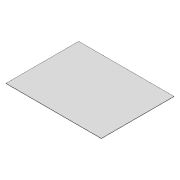
# Autodesk Inventor part: FirewallDiagonal
Saved by Autodesk Inventor 2021 (Build 250183000, 183)
## iProperties
Created: 2020-10-17
Part Number: FirewallDiagonal
Material: Generic
Document SubType Name: Modeling
Designer: PhotonUser
Density: 1 g/cm^3
Appearance: Default
Author: PhotonUser
Autodesk Inventor part; units mm, degrees
ref_plane "YZ Plane" through (0, 0, 0) normal (1, 0, 0) x (0, 1, 0)
ref_plane "XZ Plane" through (0, 0, 0) normal (0, 1, 0) x (-1, 0, 0)
ref_plane "XY Plane" through (0, 0, 0) normal (0, 0, 1) x (1, 0, 0)
sketch "Sketch1" plane through (0, 0, 0) normal (0, 1, 0) x (-1, 0, 0)
  line L0 (284.8412, -112.3127) -> (-273.9588, -112.3127)
  line L1 (-273.9588, -112.3127) -> (-273.9588, 313.8993)
  line L2 (-273.9588, 313.8993) -> (284.8412, 313.8993)
  line L3 (284.8412, 313.8993) -> (284.8412, -112.3127)
  point P0 (0, 0)
  constraints: 8 end point, 3 perpendicular, 1 horizontal
extrude "Extrusion1" add sketch "Sketch1" along normal blind 1.6002
body "Solid1"
